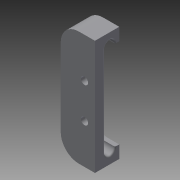
# Autodesk Inventor part: HolderFront
Saved by Autodesk Inventor 2015 (Build 190159000, 159)
## iProperties
Created: 2017-03-07
Part Number: HolderFront
Material: Generic
Document SubType Name: Modeling
Designer: 1esh9
Density: 1 g/cm^3
Appearance: Default
Author: 1esh9
Autodesk Inventor part; units mm, degrees
ref_plane "YZ Plane" through (0, 0, 0) normal (1, 0, 0) x (0, 1, 0)
ref_plane "XZ Plane" through (0, 0, 0) normal (0, 1, 0) x (-1, 0, 0)
ref_plane "XY Plane" through (0, 0, 0) normal (0, 0, 1) x (1, 0, 0)
sketch "Sketch1" plane through (0, 0, 0) normal (0, 1, 0) x (-1, 0, 0)
  circle A0 centre (0, 12.5) radius 2.6
  circle A1 centre (0, -12.5) radius 2.6
  circle A2 centre (0, 12.5) radius 4.75
  circle A3 centre (0, -12.5) radius 4.75
  circle A4 centre (0, 12.5) radius 7.5
  circle A5 centre (0, -12.5) radius 7.5
  line L0 (7.5, 12.5) -> (7.5, -12.5)
  line L1 (-7.5, -12.5) -> (-7.5, 12.5)
  line L2 (0, 12.5) -> (0, -12.5) construction
  line L3 (7.5, -12.5) -> (7.5, 12.5)
  line L4 (-7.5, 41) -> (4, 41)
  line L5 (17, 28) -> (17, -28)
  line L6 (4, -41) -> (-7.5, -41)
  line L7 (-7.5, -41) -> (-7.5, 41)
  arc A6 (4, -41) -> (17, -28) centre (4, -28) ccw
  arc A7 (17, 28) -> (4, 41) centre (4, 28) ccw
  point P0 (0, 0)
  point P1 (17, -41)
  point P2 (17, 41)
  dimension "d0" = 5.2
  dimension "d1" = 5.2
  dimension "d2" = 25
  dimension "d3" = 12.5
  dimension "d6" = 9.5
  dimension "d7" = 9.5
  dimension "d8" = 15
  dimension "d9" = 15
  dimension "d19" = 24.5
  dimension "d20" = 82
  dimension "d21" = 41
  dimension "d22" = 13
  constraints: 16 end point, 8 centre point, 8 point on circle, 7 tangent, 4 coincident, 4 point on line, 2 parallel, 1 collinear, 1 equal radius, 1 horizontal, 1 midpoint, 1 perpendicular, 1 vertical
  measures "d0" diameter of A0
  measures "d1" diameter of A1
  measures "d2" distance of A1.centre A0.centre
  measures "d3" distance of point (0, 0) A1.centre
  measures "d6" diameter of A2
  measures "d7" diameter of A3
  measures "d8" diameter of A4
  measures "d9" diameter of A5
  measures "d19" distance of point (17, -41) L6.end
  measures "d20" distance of point (17, 41) point (17, -41)
  measures "d21" distance from line of point (0, 0) L4
  measures "d22" radius of A6
extrude "Extrusion1" add sketch "Sketch1" along normal blind 3 contours A2 | A3
extrude "Extrusion2" add sketch "Sketch1" along normal blind 7 contours A4 | L0 A5 L1 A4 | A4 L7 L4 A7 L5 A6 L6 A5 L0 | A5
sketch "Sketch2" plane through (0, 7, 0) normal (0, 1, 0) x (1, 0, 0)
  circle A0 centre (0, 12.5) radius 4.75 projected
  circle A1 centre (0, -12.5) radius 4.75 projected
  line L0 (-4, -41) -> (7.5, -41) projected
  line L1 (7.5, -41) -> (7.5, 41) projected
  line L2 (7.5, 41) -> (-4, 41) projected
  arc A2 (-4, 41) -> (-17, 28) centre (-4, 28) ccw projected
  line L3 (-17, 28) -> (-17, -28) projected
  arc A3 (-17, -28) -> (-4, -41) centre (-4, -28) ccw projected
  line L4 (7.5, 41) -> (7.5, -41) projected
  line L5 (7.5, -36) -> (-2.3, -36)
  line L6 (-12, -26.3) -> (-12, 26.3)
  line L7 (7.5, 36) -> (-2.3, 36)
  arc A4 (-12, -26.3) -> (-2.3, -36) centre (-2.3, -26.3) ccw
  arc A5 (-2.3, 36) -> (-12, 26.3) centre (-2.3, 26.3) ccw
  point P0 (0, 0)
  dimension "d23" = 5
  dimension "d24" = 5
  dimension "d25" = 5
  dimension "d26" = 9.7
  constraints: 6 end point, 4 point on circle, 4 tangent, 2 centre point, 2 perpendicular, 2 point on line, 1 equal radius, 1 vertical
  measures "d23" distance between parallel lines of L6 L3
  measures "d24" distance between parallel lines of L0 L5
  measures "d25" distance between parallel lines of L2 L7
  measures "d26" radius of A4
extrude "Extrusion3" add sketch "Sketch2" along normal blind 7.4 contours A3 L3 A2 L2 L1 L7 A5 L6 A4 L5 L0
sketch "Sketch3" plane through (0, 14.4, 0) normal (0, 1, 0) x (1, 0, 0)
  line L0 (7.5, -41) -> (7.5, -36) projected
  line L1 (7.5, -36) -> (-2.3, -36) projected
  arc A0 (-12, -26.3) -> (-2.3, -36) centre (-2.3, -26.3) ccw projected
  line L2 (-12, -26.3) -> (-12, 26.3) projected
  arc A1 (-2.3, 36) -> (-12, 26.3) centre (-2.3, 26.3) ccw projected
  line L3 (-2.3, 36) -> (7.5, 36) projected
  line L4 (7.5, 36) -> (7.5, 41) projected
  line L5 (7.5, 41) -> (-4, 41) projected
  arc A2 (-4, 41) -> (-17, 28) centre (-4, 28) ccw projected
  line L6 (-17, 28) -> (-17, -28) projected
  arc A3 (-17, -28) -> (-4, -41) centre (-4, -28) ccw projected
  line L7 (-4, -41) -> (7.5, -41) projected
  line L8 (7.5, -36) -> (7.5, 36) projected
  line L9 (7.5, -32) -> (-0.75, -32)
  line L10 (7.5, 32) -> (-0.75, 32)
  line L11 (-8, -24.75) -> (-8, 24.75)
  arc A4 (-8, -24.75) -> (-0.75, -32) centre (-0.75, -24.75) ccw
  arc A5 (-0.75, 32) -> (-8, 24.75) centre (-0.75, 24.75) ccw
  line L12 (7.5, -32) -> (7.5, -36)
  line L13 (7.5, 32) -> (7.5, 36)
  point P0 (0, 0)
  dimension "d29" = 64
  dimension "d30" = 32
  dimension "d31" = 4
  dimension "d32" = 7.25
  constraints: 10 end point, 4 point on circle, 4 tangent, 3 perpendicular, 2 centre point, 2 point on line, 2 vertical, 1 equal radius
  measures "d29" distance between parallel lines of L10 L9
  measures "d30" distance from line of point (0, 0) L9
  measures "d31" distance between parallel lines of L2 L11
  measures "d32" radius of A4
extrude "Extrusion4" add sketch "Sketch3" along normal blind 3 contours L7 A3 L6 A2 L5 L4 L3 A1 L2 A0 L1 L0 | L1 A0 L2 A1 L3 L8 L10 A5 L11 A4 L9
fillet "Fillet1" radius 4 5 edges at (2.6, 7, 36) (-12, 7, 0) (-9.1589, 7, -33.1589) (2.6, 7, -36) (-9.1589, 7, 33.1589)
fillet "Fillet2" radius 4 5 edges at (-12, 14.4, 0) (-9.1589, 14.4, -33.1589) (2.6, 14.4, -36) (2.6, 14.4, 36) (-9.1589, 14.4, 33.1589)
fillet "Fillet3" radius 1 7 edges at (7.5, 14.4, 32.0226) (7.5, 13.4332, 34.6529) (7.5, 7, 0) (7.5, 8.1716, -34.8284) (7.5, 8.1716, 34.8284) (7.5, 14.4, -32.0226) (7.5, 13.4332, -34.6529)
equation "\"d3\" = 0.5 * d2"
equation "\"d21\" = 0.5 * d20"
equation "\"d30\" = 0.5 * d29"
body "Solid1"
